Autodesk Fusion 360 part; units mm, degrees
(part 2 of 2)
  line L883 (1860.1244, 644.7671) -> (1858.9352, 644.774)
  line L884 (1872.92, 643.5902) -> (1871.7772, 643.7801)
  line L885 (1868.3252, 644.2507) -> (1867.1664, 644.3744)
  line L886 (1871.7772, 643.7801) -> (1870.6305, 643.9535)
  line L887 (1846.7809, 643.9143) -> (1845.5378, 643.7348)
  line L888 (1832.6619, 640.9547) -> (1831.2332, 640.5486)
  line L889 (1844.2895, 643.5382) -> (1843.0358, 643.3245)
  line L890 (1849.2515, 644.222) -> (1848.0188, 644.0767)
  line L891 (1903.586, 631.6909) -> (1902.5272, 632.3312)
  line L892 (1834.1053, 641.3462) -> (1832.6619, 640.9547)
  line L893 (1845.5378, 643.7348) -> (1844.2895, 643.5382)
  line L894 (1887.4493, 639.6336) -> (1886.3516, 640.0353)
  line L895 (1892.8936, 637.3838) -> (1891.8104, 637.8658)
  line L896 (1791.6144, 619.6678) -> (1790.6202, 618.8287)
  line L897 (1776.1161, 603.9848) -> (1775.2917, 602.9737)
  line L898 (1828.4195, 639.6933) -> (1827.0343, 639.2443)
  line L899 (1829.8192, 640.1281) -> (1828.4195, 639.6933)
  line L900 (1785.81, 614.4711) -> (1784.8794, 613.5679)
  line L901 (1786.751, 615.3639) -> (1785.81, 614.4711)
  line L902 (1803.2987, 628.1464) -> (1802.1778, 627.4345)
  line L903 (1776.9496, 604.9867) -> (1776.1161, 603.9848)
  line L904 (1821.6348, 637.308) -> (1820.3198, 636.7893)
  line L905 (1797.8138, 624.4669) -> (1796.7521, 623.6956)
  line L906 (1820.3198, 636.7893) -> (1819.0184, 636.2571)
  line L907 (1806.7349, 630.2089) -> (1805.5772, 629.5338)
  line L908 (1831.2332, 640.5486) -> (1829.8192, 640.1281)
  line L909 (1804.4318, 628.8463) -> (1803.2987, 628.1464)
  line L910 (1819.0184, 636.2571) -> (1817.7307, 635.7114)
  line L911 (1802.1778, 627.4345) -> (1801.069, 626.7104)
  line L912 (1770.5304, 596.7173) -> (1769.7667, 595.6439)
  line L913 (1801.069, 626.7104) -> (1799.9721, 625.9744)
  line L914 (1789.6369, 617.9786) -> (1788.6643, 617.1178)
  line L915 (1779.506, 607.9354) -> (1778.6445, 606.9621)
  line L916 (1772.872, 599.8855) -> (1772.083, 598.8382)
  line L917 (1815.1956, 634.5798) -> (1813.948, 633.9942)
  line L918 (1817.7307, 635.7114) -> (1816.4564, 635.1522)
  line L919 (1811.4921, 632.7837) -> (1810.2837, 632.1591)
  line L920 (1793.6358, 621.3128) -> (1792.6196, 620.4958)
  line L921 (1769.7667, 595.6439) -> (1769.0113, 594.5621)
  line L922 (1822.9637, 637.8129) -> (1821.6348, 637.308)
  line L923 (1777.7924, 605.9791) -> (1776.9496, 604.9867)
  line L924 (1781.2577, 609.8528) -> (1780.377, 608.899)
  line L925 (1782.1482, 610.7967) -> (1781.2577, 609.8528)
  line L926 (1773.6698, 600.9239) -> (1772.872, 599.8855)
  line L927 (1772.083, 598.8382) -> (1771.3025, 597.7821)
  line L928 (1798.8871, 625.2265) -> (1797.8138, 624.4669)
  line L929 (1751.3263, 562.5225) -> (1750.1926, 559.9619)
  line L930 (1824.3065, 638.304) -> (1822.9637, 637.8129)
  line L931 (1794.6633, 622.1184) -> (1793.6358, 621.3128)
  line L932 (1767.5246, 592.3734) -> (1766.7932, 591.2667)
  line L933 (1768.2639, 593.4719) -> (1767.5246, 592.3734)
  line L934 (1716.7348, 462.5937) -> (1715.7621, 459.7727)
  line L935 (1771.3025, 597.7821) -> (1770.5304, 596.7173)
  line L936 (1737.8829, 527.7843) -> (1736.9383, 525.0069)
  line L937 (1780.377, 608.899) -> (1779.506, 607.9354)
  line L938 (1713.7806, 454.1554) -> (1712.7701, 451.3608)
  line L939 (1809.0881, 631.5217) -> (1807.9052, 630.8716)
  line L940 (1712.7701, 451.3608) -> (1711.7452, 448.5765)
  line L941 (1825.6633, 638.7811) -> (1824.3065, 638.304)
  line L942 (1763.9444, 586.7604) -> (1763.2508, 585.6144)
  line L943 (1810.2837, 632.1591) -> (1809.0881, 631.5217)
  line L944 (1796.7521, 623.6956) -> (1795.702, 622.9127)
  line L945 (1778.6445, 606.9621) -> (1777.7924, 605.9791)
  line L946 (1816.4564, 635.1522) -> (1815.1956, 634.5798)
  line L947 (1790.6202, 618.8287) -> (1789.6369, 617.9786)
  line L948 (1774.4763, 601.9534) -> (1773.6698, 600.9239)
  line L949 (1783.0486, 611.7306) -> (1782.1482, 610.7967)
  line L950 (1795.702, 622.9127) -> (1794.6633, 622.1184)
  line L951 (1775.2917, 602.9737) -> (1774.4763, 601.9534)
  line L952 (1783.9589, 612.6544) -> (1783.0486, 611.7306)
  line L953 (1769.0113, 594.5621) -> (1768.2639, 593.4719)
  line L954 (1766.7932, 591.2667) -> (1766.0695, 590.152)
  line L955 (1761.2133, 582.1316) -> (1760.5481, 580.956)
  line L956 (1711.7452, 448.5765) -> (1710.705, 445.8035)
  line L957 (1734.1516, 516.6124) -> (1733.2354, 513.7963)
  line L958 (1760.5481, 580.956) -> (1759.8897, 579.7733)
  line L959 (1724.1991, 485.3496) -> (1722.3737, 479.6408)
  line L960 (1717.6967, 465.4219) -> (1716.7348, 462.5937)
  line L961 (1749.0788, 557.3796) -> (1747.9839, 554.7766)
  line L962 (1743.776, 544.1732) -> (1742.7625, 541.4786)
  line L963 (1758.593, 577.3868) -> (1757.9544, 576.1833)
  line L964 (1738.8367, 530.5499) -> (1737.8829, 527.7843)
  line L965 (1757.9544, 576.1833) -> (1757.3221, 574.973)
  line L966 (1727.8108, 496.7675) -> (1726.0091, 491.0607)
  line L967 (1761.8854, 583.2999) -> (1761.2133, 582.1316)
  line L968 (1747.9839, 554.7766) -> (1746.907, 552.1537)
  line L969 (1707.4844, 437.5601) -> (1706.3746, 434.8402)
  line L970 (1701.7302, 424.1225) -> (1700.5135, 421.4875)
  line L971 (1752.4806, 565.0608) -> (1751.3263, 562.5225)
  line L972 (1731.4169, 508.1418) -> (1729.611, 502.4633)
  line L973 (1714.7777, 456.9597) -> (1713.7806, 454.1554)
  line L974 (1742.7625, 541.4786) -> (1741.7628, 538.7682)
  line L975 (1709.6488, 443.0425) -> (1708.5755, 440.2944)
  line L976 (1704.0951, 429.4474) -> (1702.9238, 426.776)
  line L977 (1702.9238, 426.776) -> (1701.7302, 424.1225)
  line L978 (1741.7628, 538.7682) -> (1740.7758, 536.0427)
  line L979 (1765.3536, 589.0293) -> (1764.6452, 587.8987)
  line L980 (1720.5258, 473.9409) -> (1719.5913, 471.0963)
  line L981 (1708.5755, 440.2944) -> (1707.4844, 437.5601)
  line L982 (1729.611, 502.4633) -> (1727.8108, 496.7675)
  line L983 (1745.8473, 549.5115) -> (1744.8039, 546.8511)
  line L984 (1722.3737, 479.6408) -> (1720.5258, 473.9409)
  line L985 (1764.6452, 587.8987) -> (1763.9444, 586.7604)
  line L986 (1759.8897, 579.7733) -> (1759.238, 578.5835)
  line L987 (1740.7758, 536.0427) -> (1739.8007, 533.303)
  line L988 (1759.238, 578.5835) -> (1758.593, 577.3868)
  line L989 (1705.2451, 432.1357) -> (1704.0951, 429.4474)
  line L990 (1706.3746, 434.8402) -> (1705.2451, 432.1357)
  line L991 (1710.705, 445.8035) -> (1709.6488, 443.0425)
  line L992 (1733.2354, 513.7963) -> (1731.4169, 508.1418)
  line L993 (1755.4626, 571.3028) -> (1754.8548, 570.0667)
  line L994 (1754.8548, 570.0667) -> (1754.2527, 568.8243)
  line L995 (1753.6565, 567.5757) -> (1752.4806, 565.0608)
  line L996 (1726.0091, 491.0607) -> (1724.1991, 485.3496)
  line L997 (1754.2527, 568.8243) -> (1753.6565, 567.5757)
  line L998 (1735.0735, 519.4201) -> (1734.1516, 516.6124)
  line L999 (1718.6485, 468.2563) -> (1717.6967, 465.4219)
  line L1000 (1757.3221, 574.973) -> (1756.6962, 573.7561)
  line L1001 (1763.2508, 585.6144) -> (1762.5645, 584.4609)
  line L1002 (1756.6962, 573.7561) -> (1756.0763, 572.5327)
  line L1003 (1746.907, 552.1537) -> (1745.8473, 549.5115)
  line L1004 (1744.8039, 546.8511) -> (1743.776, 544.1732)
  line L1005 (1736.9383, 525.0069) -> (1736.0021, 522.2186)
  line L1006 (1739.8007, 533.303) -> (1738.8367, 530.5499)
  line L1007 (1762.5645, 584.4609) -> (1761.8854, 583.2999)
  line L1008 (1719.5913, 471.0963) -> (1718.6485, 468.2563)
  line L1009 (1699.2728, 418.8721) -> (1698.6432, 417.5719)
  line L1010 (1694.7287, 409.8829) -> (1694.0524, 408.6211)
  line L1011 (1678.0443, 383.6406) -> (1677.1867, 382.532)
  line L1012 (1696.0603, 412.4238) -> (1695.3979, 411.1505)
  line L1013 (1645.3443, 352.7148) -> (1644.1282, 351.9178)
  line L1014 (1686.8819, 396.3434) -> (1686.1217, 395.152)
  line L1015 (1689.8423, 401.1773) -> (1689.1141, 399.9588)
  line L1016 (1682.9964, 390.4575) -> (1682.1935, 389.3022)
  line L1017 (1696.7159, 413.7027) -> (1696.0603, 412.4238)
  line L1018 (1715.7621, 459.7727) -> (1714.7777, 456.9597)
  line L1019 (1689.1141, 399.9588) -> (1688.3781, 398.7469)
  line L1020 (1678.8925, 384.7572) -> (1678.0443, 383.6406)
  line L1021 (1679.7314, 385.8818) -> (1678.8925, 384.7572)
  line L1022 (1699.8962, 420.1773) -> (1699.2728, 418.8721)
  line L1023 (1697.3648, 414.9871) -> (1696.7159, 413.7027)
  line L1024 (1691.9808, 404.8713) -> (1691.2755, 403.6336)
  line L1025 (1671.8377, 376.0551) -> (1670.9113, 375.0056)
  line L1026 (1677.1867, 382.532) -> (1676.3196, 381.4315)
  line L1027 (1692.6786, 406.1151) -> (1691.9808, 404.8713)
  line L1028 (1651.2331, 356.8678) -> (1650.0805, 356.0152)
  line L1029 (1750.1926, 559.9619) -> (1749.0788, 557.3796)
  line L1030 (1736.0021, 522.2186) -> (1735.0735, 519.4201)
  line L1031 (1756.0763, 572.5327) -> (1755.4626, 571.3028)
  line L1032 (1647.7377, 354.3428) -> (1646.5474, 353.5232)
  line L1033 (1646.5474, 353.5232) -> (1645.3443, 352.7148)
  line L1034 (1683.7906, 391.6202) -> (1682.9964, 390.4575)
  line L1035 (1668.0699, 371.911) -> (1667.1018, 370.8976)
  line L1036 (1682.1935, 389.3022) -> (1681.3818, 388.1544)
  line L1037 (1672.7539, 377.1132) -> (1671.8377, 376.0551)
  line L1038 (1700.5135, 421.4875) -> (1699.8962, 420.1773)
  line L1039 (8.0061, 961.0602) -> (7.6704, 958.3795)
  line L1040 (6.7127, 950.336) -> (6.4099, 947.6545)
  line L1041 (3.4151, 915.4688) -> (3.2185, 912.7867)
  line L1042 (9.809, 974.4593) -> (9.4318, 971.7801)
  line L1043 (0.9454, 856.5154) -> (0.9248, 853.8401)
  line L1044 (7.6704, 958.3795) -> (7.3429, 955.6985)
  line L1045 (2.3565, 899.3779) -> (2.2083, 896.6967)
  line L1046 (11.4007, 985.1721) -> (10.9903, 982.4945)
  line L1047 (3.2185, 912.7867) -> (3.0299, 910.1047)
  line L1048 (6.1154, 944.9727) -> (5.829, 942.2909)
  line L1049 (10.1944, 977.1381) -> (9.809, 974.4593)
  line L1050 (4.7656, 931.5624) -> (4.5202, 928.8801)
  line L1051 (1.936, 891.3349) -> (1.8119, 888.6544)
  line L1052 (1.8119, 888.6544) -> (1.6959, 885.9741)
  line L1053 (2.6771, 904.741) -> (2.5128, 902.0594)
  line L1054 (1.107, 867.2218) -> (1.0547, 864.5445)
  line L1055 (9.4318, 971.7801) -> (9.063, 969.1006)
  line L1056 (8.7024, 966.4207) -> (8.3501, 963.7406)
  line L1057 (11.8195, 987.8492) -> (11.4007, 985.1721)
  line L1058 (6.4099, 947.6545) -> (6.1154, 944.9727)
  line L1059 (4.5202, 928.8801) -> (4.2829, 926.1978)
  line L1060 (5.0192, 934.2446) -> (4.7656, 931.5624)
  line L1061 (2.2083, 896.6967) -> (2.0682, 894.0157)
  line L1062 (1.3115, 875.2563) -> (1.2354, 872.5777)
  line L1063 (1.0547, 864.5445) -> (1.0103, 861.8677)
  line L1064 (13.3695, 697.6318) -> (13.8064, 695.0242)
  line L1065 (1.558, 813.7854) -> (1.6626, 811.1211)
  line L1066 (0.9739, 859.1913) -> (0.9454, 856.5154)
  line L1067 (5.281, 936.9268) -> (5.0192, 934.2446)
  line L1068 (10.5882, 979.8165) -> (10.1944, 977.1381)
  line L1069 (3.6199, 918.151) -> (3.4151, 915.4688)
  line L1070 (1.4877, 880.6145) -> (1.3956, 877.9353)
  line L1071 (1.0103, 861.8677) -> (0.9739, 859.1913)
  line L1072 (12.1031, 705.4648) -> (12.5179, 702.8521)
  line L1073 (2.0682, 894.0157) -> (1.936, 891.3349)
  line L1074 (5.829, 942.2909) -> (5.5509, 939.6089)
  line L1075 (2.8494, 907.4228) -> (2.6771, 904.741)
  line L1076 (10.1402, 718.5529) -> (10.518, 715.9321)
  line L1077 (14.2506, 692.4183) -> (14.7021, 689.8142)
  line L1078 (4.2829, 926.1978) -> (4.0537, 923.5155)
  line L1079 (0.9103, 845.8173) -> (0.9212, 843.1442)
  line L1080 (0.9073, 848.491) -> (0.9103, 845.8173)
  line L1081 (1.2354, 872.5777) -> (1.1672, 869.8996)
  line L1082 (1.6959, 885.9741) -> (1.5878, 883.2942)
  line L1083 (8.3501, 963.7406) -> (8.0061, 961.0602)
  line L1084 (7.3429, 955.6985) -> (7.0237, 953.0174)
  line L1085 (15.1609, 687.2119) -> (15.6271, 684.6114)
  line L1086 (1.3721, 819.1166) -> (1.4612, 816.4506)
  line L1087 (4.1566, 771.2701) -> (4.3841, 768.6219)
  line L1088 (5.5509, 939.6089) -> (5.281, 936.9268)
  line L1089 (4.0537, 923.5155) -> (3.8327, 920.8332)
  line L1090 (7.0237, 953.0174) -> (6.7127, 950.336)
  line L1091 (2.5128, 902.0594) -> (2.3565, 899.3779)
  line L1092 (3.0299, 910.1047) -> (2.8494, 907.4228)
  line L1093 (12.2467, 990.5259) -> (11.8195, 987.8492)
  line L1094 (1.3956, 877.9353) -> (1.3115, 875.2563)
  line L1095 (10.9032, 713.3128) -> (11.2958, 710.6952)
  line L1096 (1.5878, 883.2942) -> (1.4877, 880.6145)
  line L1097 (3.8327, 920.8332) -> (3.6199, 918.151)
  line L1098 (1.1672, 869.8996) -> (1.107, 867.2218)
  line L1099 (10.9903, 982.4945) -> (10.5882, 979.8165)
  line L1100 (9.063, 969.1006) -> (8.7024, 966.4207)
  line L1101 (1676.3196, 381.4315) -> (1675.4429, 380.3393)
  line L1102 (1608.5652, 337.4685) -> (1606.5987, 336.8711)
  line L1103 (1690.5627, 402.4022) -> (1689.8423, 401.1773)
  line L1104 (1681.3818, 388.1544) -> (1680.5611, 387.0142)
  line L1105 (1652.3734, 357.7313) -> (1651.2331, 356.8678)
  line L1106 (1684.5761, 392.7903) -> (1683.7906, 391.6202)
  line L1107 (1691.2755, 403.6336) -> (1690.5627, 402.4022)
  line L1108 (1674.5564, 379.2555) -> (1673.6602, 378.1801)
  line L1109 (1687.634, 397.5418) -> (1686.8819, 396.3434)
  line L1110 (1596.5848, 334.0692) -> (1594.5469, 333.5457)
  line L1111 (1634.7047, 347.1411) -> (1632.9289, 346.3686)
  line L1112 (1618.2065, 340.6416) -> (1616.3043, 339.9821)
  line L1113 (1558.3134, 326.5025) -> (1556.0983, 326.1963)
  line L1114 (1606.5987, 336.8711) -> (1604.6199, 336.2861)
  line L1115 (1653.5014, 358.6055) -> (1652.3734, 357.7313)
  line L1116 (1594.5469, 333.5457) -> (1592.4977, 333.0344)
  line L1117 (1560.5201, 326.8206) -> (1558.3134, 326.5025)
  line L1118 (1669.9746, 373.9651) -> (1669.0275, 372.9335)
  line L1119 (1654.6173, 359.4902) -> (1653.5014, 358.6055)
  line L1120 (1666.1229, 369.8936) -> (1665.1332, 368.8989)
  line L1121 (1573.5746, 328.9804) -> (1571.4218, 328.5905)
  line L1122 (1688.3781, 398.7469) -> (1687.634, 397.5418)
  line L1123 (1673.6602, 378.1801) -> (1672.7539, 377.1132)
  line L1124 (1680.5611, 387.0142) -> (1679.7314, 385.8818)
  line L1125 (1698.6432, 417.5719) -> (1698.0072, 416.2769)
  line L1126 (1698.0072, 416.2769) -> (1697.3648, 414.9871)
  line L1127 (1586.284, 331.5738) -> (1584.1913, 331.1113)
  line L1128 (1564.9076, 327.4927) -> (1562.7182, 327.1507)
  line L1129 (1519.6567, 322.8991) -> (1517.3254, 322.7921)
  line L1130 (1669.0275, 372.9335) -> (1668.0699, 371.911)
  line L1131 (1667.1018, 370.8976) -> (1666.1229, 369.8936)
  line L1132 (1662.0982, 365.9721) -> (1661.0641, 365.0159)
  line L1133 (1693.3691, 407.3651) -> (1692.6786, 406.1151)
  line L1134 (1621.9707, 341.9981) -> (1620.0954, 341.3136)
  line L1135 (1556.0983, 326.1963) -> (1553.875, 325.9019)
  line L1136 (1661.0641, 365.0159) -> (1660.0187, 364.0696)
  line L1137 (1694.0524, 408.6211) -> (1693.3691, 407.3651)
  line L1138 (1569.2596, 328.2125) -> (1567.0882, 327.8466)
  line L1139 (1584.1913, 331.1113) -> (1582.0881, 330.6609)
  line L1140 (1670.9113, 375.0056) -> (1669.9746, 373.9651)
  line L1141 (1664.1326, 367.9136) -> (1663.121, 366.938)
  line L1142 (1675.4429, 380.3393) -> (1674.5564, 379.2555)
  line L1143 (1665.1332, 368.8989) -> (1664.1326, 367.9136)
  line L1144 (1656.8132, 361.2912) -> (1655.7212, 360.3855)
  line L1145 (1663.121, 366.938) -> (1662.0982, 365.9721)
  line L1146 (1648.9154, 355.1735) -> (1647.7377, 354.3428)
  line L1147 (1657.8933, 362.2072) -> (1656.8132, 361.2912)
  line L1148 (1631.1384, 345.6087) -> (1629.3333, 344.8614)
  line L1149 (1533.5241, 323.7842) -> (1531.2281, 323.6076)
  line L1150 (1695.3979, 411.1505) -> (1694.7287, 409.8829)
  line L1151 (1655.7212, 360.3855) -> (1654.6173, 359.4902)
  line L1152 (1650.0805, 356.0152) -> (1648.9154, 355.1735)
  line L1153 (1632.9289, 346.3686) -> (1631.1384, 345.6087)
  line L1154 (1582.0881, 330.6609) -> (1579.9747, 330.2227)
  line L1155 (1642.8992, 351.1322) -> (1641.6571, 350.3581)
  line L1156 (1685.3531, 393.9676) -> (1684.5761, 392.7903)
  line L1157 (1686.1217, 395.152) -> (1685.3531, 393.9676)
  line L1158 (1658.9618, 363.1334) -> (1657.8933, 362.2072)
  line L1159 (1660.0187, 364.0696) -> (1658.9618, 363.1334)
  line L1160 (1602.6289, 335.7134) -> (1600.626, 335.153)
  line L1161 (1577.8512, 329.7965) -> (1575.7178, 329.3824)
  line L1162 (1620.0954, 341.3136) -> (1618.2065, 340.6416)
  line L1163 (1638.2114, 348.7242) -> (1636.4656, 347.9263)
  line L1164 (1629.3333, 344.8614) -> (1627.5138, 344.1267)
  line L1165 (1498.4983, 322.3505) -> (1496.1255, 322.3467)
  line L1166 (1467.4081, 323.1821) -> (1464.9999, 323.3245)
  line L1167 (1407.1425, 330.0271) -> (1404.7478, 330.4411)
  line L1168 (1404.7478, 330.4411) -> (1402.3559, 330.8657)
  line L1169 (1486.5984, 322.445) -> (1484.2085, 322.4979)
  line L1170 (1531.2281, 323.6076) -> (1528.9258, 323.4427)
  line L1171 (1612.4604, 338.7005) -> (1610.5191, 338.0783)
  line L1172 (1488.9852, 322.4035) -> (1486.5984, 322.445)
  line L1173 (1588.3661, 332.0485) -> (1586.284, 331.5738)
  line L1174 (1553.875, 325.9019) -> (1551.6437, 325.6194)
  line L1175 (1623.8324, 342.6951) -> (1621.9707, 341.9981)
  line L1176 (1462.5902, 323.4779) -> (1460.1791, 323.6425)
  line L1177 (1469.8146, 323.0508) -> (1467.4081, 323.1821)
  line L1178 (1428.7909, 326.7816) -> (1426.379, 327.0993)
  line L1179 (1399.967, 331.3009) -> (1397.5812, 331.7466)
  line L1180 (1521.9826, 323.0176) -> (1519.6567, 322.8991)
  line L1181 (1397.5812, 331.7466) -> (1395.1986, 332.2029)
  line L1182 (1500.8672, 322.3656) -> (1498.4983, 322.3505)
  line L1183 (1452.9396, 324.2026) -> (1450.5248, 324.4113)
  line L1184 (1644.1282, 351.9178) -> (1642.8992, 351.1322)
  line L1185 (1450.5248, 324.4113) -> (1448.1096, 324.631)
  line L1186 (1627.5138, 344.1267) -> (1625.6801, 343.4046)
  line L1187 (1567.0882, 327.8466) -> (1564.9076, 327.4927)
  line L1188 (1380.9821, 335.161) -> (1378.6274, 335.6906)
  line L1189 (1549.4045, 325.3488) -> (1547.1576, 325.09)
  line L1190 (1440.8627, 325.3558) -> (1438.4473, 325.6192)
  line L1191 (1464.9999, 323.3245) -> (1462.5902, 323.4779)
  line L1192 (1426.379, 327.0993) -> (1423.9683, 327.4277)
  line L1193 (1411.9394, 329.231) -> (1409.5398, 329.6237)
  line L1194 (1392.8196, 332.6697) -> (1390.4441, 333.1471)
  line L1195 (1421.5591, 327.7669) -> (1419.1514, 328.1169)
  line L1196 (1547.1576, 325.09) -> (1544.9031, 324.843)
  line L1197 (1414.3414, 328.8489) -> (1411.9394, 329.231)
  line L1198 (1579.9747, 330.2227) -> (1577.8512, 329.7965)
  line L1199 (1514.9887, 322.6967) -> (1512.647, 322.6129)
  line L1200 (1517.3254, 322.7921) -> (1514.9887, 322.6967)
  line L1201 (1551.6437, 325.6194) -> (1549.4045, 325.3488)
  line L1202 (1590.4373, 332.5353) -> (1588.3661, 332.0485)
  line L1203 (1571.4218, 328.5905) -> (1569.2596, 328.2125)
  line L1204 (1616.3043, 339.9821) -> (1614.3889, 339.3351)
  line L1205 (1600.626, 335.153) -> (1598.6112, 334.605)
  line L1206 (1598.6112, 334.605) -> (1596.5848, 334.0692)
  line L1207 (1544.9031, 324.843) -> (1542.6414, 324.6077)
  line L1208 (1524.3029, 323.1477) -> (1521.9826, 323.0176)
  line L1209 (1636.4656, 347.9263) -> (1634.7047, 347.1411)
  line L1210 (1610.5191, 338.0783) -> (1608.5652, 337.4685)
  line L1211 (1542.6414, 324.6077) -> (1540.3724, 324.3843)
  line L1212 (1641.6571, 350.3581) -> (1639.9419, 349.5348)
  line L1213 (1491.3687, 322.3732) -> (1488.9852, 322.4035)
  line L1214 (1614.3889, 339.3351) -> (1612.4604, 338.7005)
  line L1215 (1526.6173, 323.2894) -> (1524.3029, 323.1477)
  line L1216 (1592.4977, 333.0344) -> (1590.4373, 332.5353)
  line L1217 (1540.3724, 324.3843) -> (1538.0964, 324.1725)
  line L1218 (1535.8136, 323.9725) -> (1533.5241, 323.7842)
  line L1219 (1639.9419, 349.5348) -> (1638.2114, 348.7242)
  line L1220 (1538.0964, 324.1725) -> (1535.8136, 323.9725)
  line L1221 (1562.7182, 327.1507) -> (1560.5201, 326.8206)
  line L1222 (1402.3559, 330.8657) -> (1399.967, 331.3009)
  line L1223 (1433.6177, 326.1787) -> (1431.2038, 326.4748)
  line L1224 (1528.9258, 323.4427) -> (1526.6173, 323.2894)
  line L1225 (1575.7178, 329.3824) -> (1573.5746, 328.9804)
  line L1226 (1455.3536, 324.0049) -> (1452.9396, 324.2026)
  line L1227 (1625.6801, 343.4046) -> (1623.8324, 342.6951)
  line L1228 (1604.6199, 336.2861) -> (1602.6289, 335.7134)
  line L1229 (1364.603, 339.0853) -> (1362.2845, 339.6871)
  line L1230 (1419.1514, 328.1169) -> (1416.7454, 328.4775)
  line L1231 (1366.9271, 338.4937) -> (1364.603, 339.0853)
  line L1232 (1510.3002, 322.5405) -> (1507.9487, 322.4796)
  line L1233 (1423.9683, 327.4277) -> (1421.5591, 327.7669)
  line L1234 (1385.7048, 334.1332) -> (1383.3413, 334.6419)
  line L1235 (1512.647, 322.6129) -> (1510.3002, 322.5405)
  line L1236 (1445.6941, 324.8617) -> (1443.2784, 325.1033)
  line L1237 (1505.5926, 322.4302) -> (1503.232, 322.3922)
  line L1238 (1507.9487, 322.4796) -> (1505.5926, 322.4302)
  line L1239 (1264.7553, 378.1225) -> (1262.8979, 379.1843)
  line L1240 (1255.6094, 383.5243) -> (1253.8234, 384.6324)
  line L1241 (1388.0725, 333.6349) -> (1385.7048, 334.1332)
  line L1242 (1245.1187, 390.3106) -> (1243.424, 391.4737)
  line L1243 (1376.2773, 336.2305) -> (1373.9321, 336.7808)
  line L1244 (1448.1096, 324.631) -> (1445.6941, 324.8617)
  line L1245 (1373.9321, 336.7808) -> (1371.5919, 337.3414)
  line L1246 (1288.0679, 366.1145) -> (1286.0567, 367.063)
  line L1247 (1493.7489, 322.3543) -> (1491.3687, 322.3732)
  line L1248 (1371.5919, 337.3414) -> (1369.2568, 337.9124)
  line L1249 (1472.2192, 322.9307) -> (1469.8146, 323.0508)
  line L1250 (1337.2059, 346.979) -> (1334.9691, 347.7024)
  line L1251 (1346.2289, 344.1856) -> (1343.9621, 344.8688)
  line L1252 (1296.2278, 362.4162) -> (1294.1708, 363.3263)
  line L1253 (1266.6264, 377.0701) -> (1264.7553, 378.1225)
  line L1254 (1484.2085, 322.4979) -> (1481.8157, 322.562)
  line L1255 (1262.8979, 379.1843) -> (1261.0545, 380.2554)
  line L1256 (1261.0545, 380.2554) -> (1259.2251, 381.3357)
  line L1257 (1268.5111, 376.027) -> (1266.6264, 377.0701)
  line L1258 (1362.2845, 339.6871) -> (1359.9719, 340.2992)
  line L1259 (1383.3413, 334.6419) -> (1380.9821, 335.161)
  line L1260 (1294.1708, 363.3263) -> (1292.1251, 364.2461)
  line L1261 (1246.829, 389.1567) -> (1245.1187, 390.3106)
  line L1262 (1286.0567, 367.063) -> (1284.0574, 368.0211)
  line L1263 (1259.2251, 381.3357) -> (1257.41, 382.4254)
  line L1264 (1257.41, 382.4254) -> (1255.6094, 383.5243)
  line L1265 (1250.2959, 386.8762) -> (1248.5548, 388.0119)
  line L1266 (1272.3206, 373.9689) -> (1270.4093, 374.9932)
  line L1267 (1350.7834, 342.8495) -> (1348.5027, 343.5125)
  line L1268 (1460.1791, 323.6425) -> (1457.7669, 323.8182)
  line L1269 (1416.7454, 328.4775) -> (1414.3414, 328.8489)
  line L1270 (1395.1986, 332.2029) -> (1392.8196, 332.6697)
  line L1271 (1238.4355, 395.0173) -> (1236.8051, 396.2165)
  line L1272 (1409.5398, 329.6237) -> (1407.1425, 330.0271)
  line L1273 (1343.9621, 344.8688) -> (1341.7026, 345.5622)
  line L1274 (1443.2784, 325.1033) -> (1440.8627, 325.3558)
  line L1275 (1496.1255, 322.3467) -> (1493.7489, 322.3543)
  line L1276 (1457.7669, 323.8182) -> (1455.3536, 324.0049)
  line L1277 (1369.2568, 337.9124) -> (1366.9271, 338.4937)
  line L1278 (1436.0322, 325.8935) -> (1433.6177, 326.1787)
  line L1279 (1378.6274, 335.6906) -> (1376.2773, 336.2305)
  line L1280 (1270.4093, 374.9932) -> (1268.5111, 376.027)
  line L1281 (1477.0222, 322.7239) -> (1474.6218, 322.8217)
  line L1282 (1438.4473, 325.6192) -> (1436.0322, 325.8935)
  line L1283 (1334.9691, 347.7024) -> (1332.7402, 348.4359)
  line L1284 (1300.3745, 360.6249) -> (1298.2957, 361.5157)
  line L1285 (1328.3069, 349.9327) -> (1326.1028, 350.6961)
  line L1286 (1280.0952, 369.9658) -> (1278.1325, 370.9524)
  line L1287 (1479.4203, 322.6374) -> (1477.0222, 322.7239)
  line L1288 (1481.8157, 322.562) -> (1479.4203, 322.6374)
  line L1289 (1431.2038, 326.4748) -> (1428.7909, 326.7816)
  line L1290 (1503.232, 322.3922) -> (1500.8672, 322.3656)
  line L1291 (1474.6218, 322.8217) -> (1472.2192, 322.9307)
  line L1292 (1390.4441, 333.1471) -> (1388.0725, 333.6349)
  line L1293 (1233.594, 398.6421) -> (1232.0136, 399.8684)
  line L1294 (1321.7206, 352.2526) -> (1319.5429, 353.0456)
  line L1295 (1348.5027, 343.5125) -> (1346.2289, 344.1856)
  line L1296 (1332.7402, 348.4359) -> (1330.5194, 349.1793)
  line L1297 (1310.9249, 356.3164) -> (1308.7945, 357.1586)
  line L1298 (1330.5194, 349.1793) -> (1328.3069, 349.9327)
  line L1299 (1252.0522, 385.7497) -> (1250.2959, 386.8762)
  line L1300 (1326.1028, 350.6961) -> (1323.9073, 351.4694)
  line L1301 (1315.215, 354.6613) -> (1313.0651, 355.484)
  line L1302 (1240.0822, 393.827) -> (1238.4355, 395.0173)
  line L1303 (1235.1912, 397.4248) -> (1233.594, 398.6421)
  line L1304 (1357.6653, 340.9215) -> (1355.3649, 341.554)
  line L1305 (1248.5548, 388.0119) -> (1246.829, 389.1567)
  line L1306 (1276.1825, 371.9484) -> (1274.2451, 372.954)
  line L1307 (1353.0709, 342.1966) -> (1350.7834, 342.8495)
  line L1308 (1341.7026, 345.5622) -> (1339.4504, 346.2655)
  line L1309 (1236.8051, 396.2165) -> (1235.1912, 397.4248)
  line L1310 (1253.8234, 384.6324) -> (1252.0522, 385.7497)
  line L1311 (1359.9719, 340.2992) -> (1357.6653, 340.9215)
  line L1312 (1323.9073, 351.4694) -> (1321.7206, 352.2526)
  line L1313 (1241.7451, 392.6458) -> (1240.0822, 393.827)
  line L1314 (1302.4639, 359.7437) -> (1300.3745, 360.6249)
  line L1315 (1308.7945, 357.1586) -> (1306.6741, 358.0105)
  line L1316 (1339.4504, 346.2655) -> (1337.2059, 346.979)
  line L1317 (1355.3649, 341.554) -> (1353.0709, 342.1966)
  line L1318 (1317.3743, 353.8486) -> (1315.215, 354.6613)
  line L1319 (1319.5429, 353.0456) -> (1317.3743, 353.8486)
  line L1320 (1306.6741, 358.0105) -> (1304.5638, 358.8723)
  line L1321 (1304.5638, 358.8723) -> (1302.4639, 359.7437)
  line L1322 (1290.0907, 365.1755) -> (1288.0679, 366.1145)
  line L1323 (1292.1251, 364.2461) -> (1290.0907, 365.1755)
  line L1324 (1243.424, 391.4737) -> (1241.7451, 392.6458)
  line L1325 (1181.1192, 464.007) -> (1180.4994, 465.6242)
  line L1326 (1298.2957, 361.5157) -> (1296.2278, 362.4162)
  line L1327 (1183.1262, 459.2039) -> (1182.4328, 460.7969)
  line L1328 (1192.3159, 442.2209) -> (1191.3654, 443.7236)
  line L1329 (1184.5857, 456.0423) -> (1183.844, 457.6191)
  line L1330 (1199.5859, 431.9366) -> (1198.4825, 433.3805)
  line L1331 (1210.4468, 419.3245) -> (1209.1593, 420.6916)
  line L1332 (1209.1593, 420.6916) -> (1207.8917, 422.0672)
  line L1333 (1230.4503, 401.1035) -> (1228.9041, 402.3477)
  line L1334 (1178.2713, 472.173) -> (1177.7778, 473.8301)
  line L1335 (1177.7778, 473.8301) -> (1177.3101, 475.4952)
  line L1336 (1176.0634, 480.5377) -> (1175.7005, 482.2342)
  line L1337 (1219.9979, 409.9987) -> (1218.5769, 411.3048)
  line L1338 (1183.844, 457.6191) -> (1183.1262, 459.2039)
  line L1339 (1178.7903, 470.5238) -> (1178.2713, 472.173)
  line L1340 (1175.7005, 482.2342) -> (1175.3643, 483.9386)
  line L1341 (1175.3643, 483.9386) -> (1175.0549, 485.6508)
  line L1342 (1224.3706, 406.1334) -> (1222.8949, 407.413)
  line L1343 (1193.2888, 440.7266) -> (1192.3159, 442.2209)
  line L1344 (1187.7899, 449.8171) -> (1186.9537, 451.3611)
  line L1345 (1177.3101, 475.4952) -> (1176.8684, 477.1681)
  line L1346 (1186.9537, 451.3611) -> (1186.1407, 452.9133)
  line L1347 (1174.7724, 487.3708) -> (1174.5171, 489.0986)
  line L1348 (1176.4527, 478.849) -> (1176.0634, 480.5377)
  line L1349 (1179.9046, 467.2494) -> (1179.3348, 468.8826)
  line L1350 (1194.2839, 439.2406) -> (1193.2888, 440.7266)
  line L1351 (1188.6494, 448.2813) -> (1187.7899, 449.8171)
  line L1352 (1198.4825, 433.3805) -> (1197.4005, 434.8329)
  line L1353 (1196.3399, 436.2937) -> (1195.301, 437.763)
  line L1354 (1174.2891, 490.8341) -> (1174.0886, 492.5773)
  line L1355 (1214.426, 415.2755) -> (1213.0803, 416.6165)
  line L1356 (1213.0803, 416.6165) -> (1211.7538, 417.9662)
  line L1357 (1207.8917, 422.0672) -> (1206.6439, 423.4514)
  line L1358 (1186.1407, 452.9133) -> (1185.3514, 454.4738)
  line L1359 (1180.4994, 465.6242) -> (1179.9046, 467.2494)
  line L1360 (1203.0221, 427.6556) -> (1201.8558, 429.0741)
  line L1361 (1175.0549, 485.6508) -> (1174.7724, 487.3708)
  line L1362 (1174.0886, 492.5773) -> (1173.9158, 494.3283)
  line L1363 (1173.9158, 494.3283) -> (1173.7708, 496.0869)
  line L1364 (1228.9041, 402.3477) -> (1227.3753, 403.6007)
  line L1365 (1232.0136, 399.8684) -> (1230.4503, 401.1035)
  line L1366 (1181.7637, 462.3979) -> (1181.1192, 464.007)
  line L1367 (1197.4005, 434.8329) -> (1196.3399, 436.2937)
  line L1368 (1217.1745, 412.6196) -> (1215.7908, 413.9432)
  line L1369 (1218.5769, 411.3048) -> (1217.1745, 412.6196)
  line L1370 (1313.0651, 355.484) -> (1310.9249, 356.3164)
  line L1371 (1195.301, 437.763) -> (1194.2839, 439.2406)
  line L1372 (1284.0574, 368.0211) -> (1282.0702, 368.9887)
  line L1373 (1278.1325, 370.9524) -> (1276.1825, 371.9484)
  line L1374 (1274.2451, 372.954) -> (1272.3206, 373.9689)
  line L1375 (1179.3348, 468.8826) -> (1178.7903, 470.5238)
  line L1376 (1282.0702, 368.9887) -> (1280.0952, 369.9658)
  line L1377 (1215.7908, 413.9432) -> (1214.426, 415.2755)
  line L1378 (1205.4163, 424.8443) -> (1204.209, 426.2457)
  line L1379 (1191.3654, 443.7236) -> (1190.4373, 445.2345)
  line L1380 (1222.8949, 407.413) -> (1221.4373, 408.7015)
  line L1381 (1221.4373, 408.7015) -> (1219.9979, 409.9987)
  line L1382 (1201.8558, 429.0741) -> (1200.7104, 430.5011)
  line L1383 (1206.6439, 423.4514) -> (1205.4163, 424.8443)
  line L1384 (1185.3514, 454.4738) -> (1184.5857, 456.0423)
  line L1385 (1190.4373, 445.2345) -> (1189.5319, 446.7538)
  line L1386 (1200.7104, 430.5011) -> (1199.5859, 431.9366)
  line L1387 (1176.8684, 477.1681) -> (1176.4527, 478.849)
  line L1388 (1211.7538, 417.9662) -> (1210.4468, 419.3245)
  line L1389 (146.7071, 990.7854) -> (119.8159, 990.7066)
  line L1390 (711.3855, 991.8363) -> (684.4954, 991.9419)
  line L1391 (388.715, 991.7098) -> (334.9369, 991.5054)
  line L1392 (818.9493, 991.104) -> (805.5035, 991.225)
  line L1393 (603.8266, 992.1024) -> (576.9373, 992.11)
  line L1394 (1168.4758, 635.0939) -> (872.9542, 635.0939)
  line L1395 (334.9369, 991.5054) -> (281.1582, 991.288)
  line L1396 (872.7337, 745.9006) -> (872.7337, 990.5259)
  line L1397 (496.2704, 992.0208) -> (469.3816, 991.9599)
  line L1398 (39.1397, 990.5473) -> (12.2467, 990.5259)
  line L1399 (1173.565, 499.6272) -> (1173.4424, 502.3508)
  line L1400 (859.2874, 990.685) -> (845.8413, 990.8341)
  line L1401 (684.4954, 991.9419) -> (657.6056, 992.0202)
  line L1402 (1174.5171, 489.0986) -> (1174.2891, 490.8341)
  line L1403 (1204.209, 426.2457) -> (1203.0221, 427.6556)
  line L1404 (1173.6538, 497.8532) -> (1173.565, 499.6272)
  line L1405 (415.6039, 991.8026) -> (388.715, 991.7098)
  line L1406 (1173.2385, 507.3503) -> (1172.6344, 522.8827)
  line L1407 (1189.5319, 446.7538) -> (1188.6494, 448.2813)
  line L1408 (751.7213, 991.6227) -> (738.2759, 991.7016)
  line L1409 (872.9542, 745.5218) -> (872.7337, 745.9006)
  line L1410 (738.2759, 991.7016) -> (711.3855, 991.8363)
  line L1411 (469.3816, 991.9599) -> (442.4927, 991.8866)
  line L1412 (576.9373, 992.11) -> (550.0483, 992.0977)
  line L1413 (92.9243, 990.6394) -> (66.0323, 990.5857)
  line L1414 (1170.9717, 567.02) -> (1169.3333, 611.3276)
  line L1415 (832.3953, 990.9737) -> (818.9493, 991.104)
  line L1416 (1172.6344, 522.8827) -> (1171.8473, 543.6356)
  line L1417 (442.4927, 991.8866) -> (415.6039, 991.8026)
  line L1418 (1225.8641, 404.8626) -> (1224.3706, 406.1334)
  line L1419 (792.0578, 991.3372) -> (778.6122, 991.4407)
  line L1420 (550.0483, 992.0977) -> (523.1593, 992.0673)
  line L1421 (523.1593, 992.0673) -> (496.2704, 992.0208)
  line L1422 (872.9542, 635.0939) -> (872.9542, 745.5218)
  line L1423 (1168.7596, 627.0729) -> (1168.4758, 635.0939)
  line L1424 (1173.4424, 502.3508) -> (1173.2385, 507.3503)
  line L1425 (765.1667, 991.5358) -> (751.7213, 991.6227)
  line L1426 (1169.3333, 611.3276) -> (1168.7596, 627.0729)
  line L1427 (1227.3753, 403.6007) -> (1225.8641, 404.8626)
  line L1428 (1171.8473, 543.6356) -> (1170.9717, 567.02)
  line L1429 (119.8159, 990.7066) -> (92.9243, 990.6394)
  line L1430 (657.6056, 992.0202) -> (630.7159, 992.0731)
  line L1431 (281.1582, 991.288) -> (227.3786, 991.0726)
  line L1432 (630.7159, 992.0731) -> (603.8266, 992.1024)
  line L1433 (1182.4328, 460.7969) -> (1181.7637, 462.3979)
  line L1434 (66.0323, 990.5857) -> (39.1397, 990.5473)
  line L1435 (845.8413, 990.8341) -> (832.3953, 990.9737)
  line L1436 (173.598, 990.8738) -> (146.7071, 990.7854)
  line L1437 (872.7337, 990.5259) -> (859.2874, 990.685)
  line L1438 (1173.7708, 496.0869) -> (1173.6538, 497.8532)
  line L1439 (227.3786, 991.0726) -> (173.598, 990.8738)
  line L1440 (778.6122, 991.4407) -> (765.1667, 991.5358)
  line L1441 (805.5035, 991.225) -> (792.0578, 991.3372)
extrude "Extrude1" add sketch "export_vcarve" along normal blind 12 makes body 1 in component "hlid_1"
sketch "Sketch1" plane through (0, 0, 0) normal (0, 0, 1) x (1, 0, 0)
box "BoxPrimitive1" add length 1100 width 1200 height 12 placed x (0, 1, 0) y (-1, 0, 0) z (0, 0, 1) at (1200, 800, 0) separate body makes body 2 in component "botn_plata"
copy_body "CopyPasteBodies1" bodies 2 makes body 3 in component "botn_plata"
move_body "Move1" bodies 3 to x (1, 0, 0) y (0, 1, 0) z (0, 0, 1) at (0, 1600, 0) in component "botn_plata"
move_face "OffsetFaces1" offset -750 1 faces at (800, 3500, 4) on bodies 3 in component "botn_plata"
move_body "Move2" bodies 3 to x (1, 0, 0) y (0, 0, 1) z (0, -1, 0) at (0, 180.8692, -1804.1771) in component "botn_plata"
copy_body "CopyPasteBodies2" bodies 3 makes body 4 in component "botn_plata"
move_body "Move3" bodies 4 to x (1, 0, 0) y (0, 1, 0) z (0, 0, 1) at (0, 0, 700) in component "botn_plata"
move_face "OffsetFaces2" offset 10 1 faces at (400, 176.8692, 1645.8229) on bodies 4 in component "botn_plata"
copy_body "CopyPasteBodies3" bodies 4 makes body 5 in component "botn_plata"
move_body "Move4" bodies 5 to x (1, 0, 0) y (0, 1, 0) z (0, 0, 1) at (0, 0, 650) in component "botn_plata"
move_face "OffsetFaces3" offset -40 1 faces at (400, 176.8692, 2305.8229) on bodies 5 in component "botn_plata"
move_body "Move5" bodies 4 to x (1, 0, 0) y (0, 0.5, 0.866025) z (0, -0.866025, 0.5) at (0, 1819.0182, -791.7456) in component "botn_plata"
move_body "Move6" bodies 5 to x (1, 0, 0) y (0, 0.819152, 0.573576) z (0, -0.573576, 0.819152) at (0, 1374.1675, -1449.7467) in component "botn_plata"
copy_body "CopyPasteBodies4" bodies 3 makes body 6 in component "botn_plata"
move_body "Move7" bodies 6 to x (1, 0, 0) y (0, 1, 0) z (0, 0, 1) at (0, 1050, 0) in component "botn_plata"
move_face "OffsetFaces4" offset 100 1 faces at (400, 1226.8692, 945.8229) on bodies 6 in component "botn_plata"
copy_body "CopyPasteBodies5" bodies 6 makes body 7 in component "botn_plata"
move_body "Move8" bodies 7 to x (1, 0, 0) y (0, 0, -1) z (0, 1, 0) at (0, 923.0463, 1814.6921) in component "botn_plata"
move_face "OffsetFaces5" offset 10 1 faces at (400, 1968.8692, 587.8229) on bodies 7 in component "botn_plata"
copy_body "CopyPasteBodies6" bodies 6 makes body 8 in component "botn_plata"
move_body "Move9" bodies 8 to x (1, 0, 0) y (0, 1, 0) z (0, 0, 1) at (0, -250, 0) in component "botn_plata"
move_body "Move10" bodies 6 to x (1, 0, 0) y (0, 1, 0) z (0, 0, 1) at (0, 0, -580) in component "botn_plata"
move_body "Move11" bodies 6 to x (1, 0, 0) y (0, 1, 0) z (0, 0, 1) at (0, 0, -4) in component "botn_plata"
move_body "Move12" bodies 8 to x (1, 0, 0) y (0, 1, 0) z (0, 0, 1) at (0, -14.9074, -132.5099) in component "botn_plata"
move_body "Move13" bodies 7 to x (1, 0, 0) y (0, 1, 0) z (0, 0, 1) at (0, -708.5028, -121.0426) in component "botn_plata"
move_body "Move14" bodies 8 to x (1, 0, 0) y (0, 1, 0) z (0, 0, 1) at (0, -137.6545, 9.5299) in component "botn_plata"
move_body "Move15" bodies 4 to x (1, 0, 0) y (0, 1, 0) z (0, 0, 1) at (0, 9.284, -0.6473) in component "botn_plata"
copy_body "CopyPasteBodies7" bodies 7 makes body 9 in component "botn_plata"
move_body "Move16" bodies 9 to x (1, 0, 0) y (0, 1, 0) z (0, 0, 1) at (0, 850, 0) in component "botn_plata"
move_face "OffsetFaces6" offset -70 1 faces at (400, 2120.3664, 466.7803) on bodies 9 in component "botn_plata"
copy_body "CopyPasteBodies8" bodies 9 makes body 10 in component "botn_plata"
move_body "Move17" bodies 10 to x (1, 0, 0) y (0, 1, 0) z (0, 0, 1) at (0, 750, 0) in component "botn_plata"
move_face "OffsetFaces7" offset 130 1 faces at (400, 2800.3664, 466.7803) on bodies 10 in component "botn_plata"
copy_body "CopyPasteBodies9" bodies 10 makes body 11 in component "botn_plata"
move_body "Move18" bodies 11 to x (1, 0, 0) y (0, 1, 0) z (0, 0, 1) at (0, 800, 0) in component "botn_plata"
move_face "OffsetFaces8" offset -350 1 faces at (400, 3730.3664, 466.7803) on bodies 11 in component "botn_plata"
move_body "Move19" bodies 9 to x (1, 0, 0) y (0, 0.939693, 0.34202) z (0, -0.34202, 0.939693) at (0, 477.8409, -994.0286) in component "botn_plata"
move_body "Move20" bodies 11 to x (1, 0, 0) y (0, 1, 0) z (0, 0, 1) at (0, -1336.6347, 87.9365) in component "botn_plata"
move_body "Move21" bodies 10 to x (1, 0, 0) y (0, -0.5, 0.866025) z (0, -0.866025, -0.5) at (0, 3865.1975, -1702.0732) in component "botn_plata"
move_body "Move22" bodies 11 to x (1, 0, 0) y (0, 1, 0) z (0, 0, 1) at (0, -20.1966, -34.5025) in component "botn_plata"
move_body "Move23" bodies 2 to x (1, 0, 0) y (0, 1, 0) z (0, 0, 1) at (0, -25, 0) in component "botn_plata"
move_body "Move24" bodies 4 to x (1, 0, 0) y (0, 1, 0) z (0, 0, 1) at (0, -21.8796, 2.5246) in component "botn_plata"
move_body "Move25" bodies 5 to x (1, 0, 0) y (0, 0.984808, 0.173648) z (0, -0.173648, 0.984808) at (0, 103.05, -117.2075) in component "botn_plata"
move_body "Move26" bodies 3 to x (1, 0, 0) y (0, 0.965926, 0.258819) z (0, -0.258819, 0.965926) at (0, 209.9293, -196.2655) in component "botn_plata"
move_body "Move27" bodies 8 to x (1, 0, 0) y (0, 1, 0) z (0, 0, 1) at (0, -5.9409, 1.9373) in component "botn_plata"
component "hlid_1" placed x (1, 0, 0) y (0, 1, 0) z (0, 0, 1) at (-12, 0, 0)
component "hlid_1" placed x (1, 0, 0) y (0, 1, 0) z (0, 0, 1) at (1200, 0, 0)
component "botn_plata" placed x (1, 0, 0) y (0, 1, 0) z (0, 0, 1) at (0, -100, 25)
component "sæti" placed x (1, 0, 0) y (0, 1, 0) z (0, 0, 1) at (0, 0, 0)
equation "d1 = thi_platta"
equation "thi_platta = 12 mm"
equation "plötu_breidd = 1200 mm"
equation "botn_lengd = 1100 mm"
equation "d8 = thi_platta"
named bodies: "botn_plata", "efra_bak", "neðra_bak (1)", "mið_bak (1) (1)", "efra_bak (1)", "uppstig (1)", "framstig (1) (1)", "uppstig (1) (1)", "neðrifesting (1) (1) (1)", "fremri festing (1) (1) (1) (1)", "festing ofan"
